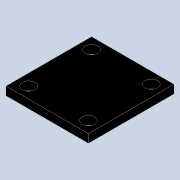
# Autodesk Inventor part: Y Axis Belt Stationary Top
Saved by Autodesk Inventor 2022 (Build 260153000, 153)
## iProperties
Created: 2021-10-19
Part Number: Y Axis Belt Stationary Top
Material: Generic
Document SubType Name: Modeling
Designer: Coy
Density: 1 g/cm^3
Appearance: Anodized - Black
Author: Coy
Autodesk Inventor part; units mm, degrees
ref_plane "YZ Plane" through (0, 0, 0) normal (1, 0, 0) x (0, 1, 0)
ref_plane "XZ Plane" through (0, 0, 0) normal (0, 1, 0) x (-1, 0, 0)
ref_plane "XY Plane" through (0, 0, 0) normal (0, 0, 1) x (1, 0, 0)
sketch "Sketch1" plane through (0, 0, 0) normal (0, 1, 0) x (-1, 0, 0)
  circle A0 centre (29.4, 55.3) radius 2.6
  circle A1 centre (4.7, 55.3) radius 2.6
  line L0 (34.1, 50.3) -> (34.1, 60)
  line L1 (34.1, 60) -> (0, 60)
  line L2 (0, 60) -> (0, 50.3)
  circle A2 centre (29.4, 29.3) radius 2.6
  circle A3 centre (4.7, 29.3) radius 2.6
  line L3 (0, 34.3) -> (0, 24.6)
  line L4 (0, 24.6) -> (34.1, 24.6)
  line L5 (34.1, 24.6) -> (34.1, 34.3)
  line L6 (34.1, 50.3) -> (34.1, 34.3)
  line L7 (0, 50.3) -> (0, 34.3)
  point P0 (0, 0)
  point P1 (0, 0)
  constraints: 16 end point, 4 centre point
extrude "Extrusion1" add sketch "Sketch1" along normal blind 3.5
body "Solid1"
